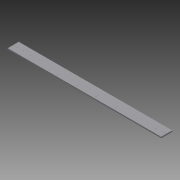
# Autodesk Inventor part: licht_50
Saved by Autodesk Inventor 2015 (Build 190159000, 159)
## iProperties
Created: 2018-01-11
Part Number: licht_50
Material: Generisch
Document SubType Name: Modeling
Designer: schueler
Density: 1 g/cm^3
Appearance: Vorgabe
Author: schueler
Autodesk Inventor part; units mm, degrees
ref_plane "YZ Plane" through (0, 0, 0) normal (1, 0, 0) x (0, 1, 0)
ref_plane "XZ Plane" through (0, 0, 0) normal (0, 1, 0) x (-1, 0, 0)
ref_plane "XY Plane" through (0, 0, 0) normal (0, 0, 1) x (1, 0, 0)
sketch "Skizze1" plane through (0, 0, 0) normal (0, 0, 1) x (1, 0, 0)
  line L0 (0, 0) -> (2000, 0)
  line L1 (2000, 0) -> (2000, 144)
  line L2 (2000, 144) -> (0, 144)
  line L3 (0, 144) -> (0, 0)
  line L4 (0, 25) -> (2000, 25) construction
  line L5 (0, 50) -> (2000, 50) construction
  line L6 (1000, 0) -> (1000, 144) construction
  line L7 (875, 0) -> (875, 144) construction
  line L8 (1125, 144) -> (1125, 0) construction
  line L9 (1375, 144) -> (1375, 0) construction
  line L10 (625, 144) -> (625, 0) construction
  circle A0 centre (625, 50) radius 2.5
  circle A1 centre (875, 50) radius 2.5
  circle A2 centre (1125, 50) radius 2.5
  circle A3 centre (1375, 50) radius 2.5
  circle A4 centre (1375, 25) radius 3.5
  circle A5 centre (1125, 25) radius 3.5
  circle A6 centre (875, 25) radius 3.5
  circle A7 centre (625, 25) radius 3.5
  line L11 (50, 144) -> (50, 0) construction
  circle A8 centre (50, 72) radius 4
  line L12 (1950, 144) -> (1950, 0) construction
  circle A9 centre (1950, 72) radius 4
  line L13 (1992, 144) -> (1992, 0) construction
  line L14 (2000, 112) -> (0, 112) construction
  line L15 (2000, 32) -> (0, 32) construction
  circle A10 centre (1992, 112) radius 1.5
  circle A11 centre (1992, 32) radius 1.5
  line L16 (8, 144) -> (8, 0) construction
  circle A12 centre (8, 112) radius 1.5
  circle A13 centre (8, 72) radius 1.5
  circle A14 centre (8, 32) radius 1.5
  circle A15 centre (1992, 72) radius 1.5
  circle A16 centre (1000, 72) radius 1.5
  circle A17 centre (1000, 112) radius 1.5
  circle A18 centre (1000, 32) radius 1.5
  circle A19 centre (1870, 62) radius 1.5
  circle A20 centre (1970, 72) radius 1.5
  circle A21 centre (1870, 82) radius 1.5
  circle A22 centre (1670, 82) radius 1.5
  circle A23 centre (1670, 62) radius 1.5
  circle A24 centre (1770, 72) radius 1.5
  line L17 (2000, 72) -> (1650, 72) construction
  line L18 (1870, 82) -> (1670, 82) construction
  line L19 (1670, 82) -> (1670, 62) construction
  line L20 (1670, 62) -> (1870, 62) construction
  line L21 (1870, 62) -> (1870, 82) construction
  line L22 (0, 72) -> (350, 72) construction
  circle A25 centre (30, 72) radius 1.5
  circle A26 centre (130, 82) radius 1.5
  circle A27 centre (130, 62) radius 1.5
  circle A28 centre (230, 72) radius 1.5
  circle A29 centre (330, 82) radius 1.5
  circle A30 centre (330, 62) radius 1.5
  line L23 (130, 82) -> (330, 82) construction
  line L24 (330, 82) -> (330, 62) construction
  line L25 (330, 62) -> (130, 62) construction
  line L26 (130, 62) -> (130, 82) construction
  dimension "d0" = 2000
  dimension "d1" = 144
  dimension "d2" = 25
  dimension "d3" = 50
  dimension "d4" = 125
  dimension "d5" = 125
  dimension "d6" = 250
  dimension "d7" = 250
  dimension "d8" = 5
  dimension "d9" = 5
  dimension "d10" = 5
  dimension "d11" = 5
  dimension "d12" = 7
  dimension "d13" = 7
  dimension "d14" = 7
  dimension "d15" = 7
  dimension "d16" = 50
  dimension "d17" = 8
  dimension "d18" = 50
  dimension "d19" = 8
  dimension "d20" = 8
  dimension "d21" = 40
  dimension "d22" = 40
  dimension "d23" = 3
  dimension "d24" = 3
  dimension "d25" = 8
  dimension "d26" = 3
  dimension "d27" = 3
  dimension "d28" = 3
  dimension "d29" = 3
  dimension "d30" = 3
  dimension "d31" = 3
  dimension "d32" = 3
  dimension "d137" = 3
  dimension "d138" = 3
  dimension "d139" = 3
  dimension "d141" = 3
  dimension "d142" = 3
  dimension "d143" = 3
  dimension "d144" = 350
  dimension "d145" = 30
  dimension "d146" = 100
  dimension "d147" = 100
  dimension "d148" = 100
  dimension "d149" = 10
  dimension "d150" = 10
  dimension "d151" = 350
  dimension "d152" = 3
  dimension "d153" = 3
  dimension "d154" = 3
  dimension "d155" = 3
  dimension "d156" = 3
  dimension "d157" = 3
  dimension "d158" = 30
  dimension "d159" = 100
  dimension "d160" = 100
  dimension "d161" = 100
  dimension "d162" = 10
  dimension "d163" = 10
  constraints: 50 end point, 38 point on line, 31 centre point, 9 midpoint, 9 vertical, 6 coincident, 6 parallel, 5 perpendicular, 4 horizontal, 24 other
  measures "d0" distance of L3.start L1.end
  measures "d1" distance of L1.end L1.start
  measures "d2" distance of L1.start L4.end
  measures "d3" distance of L1.start L5.end
  measures "d4" distance of L8.start L6.end
  measures "d5" distance of L7.end L6.end
  measures "d6" distance of L9.start L8.start
  measures "d7" distance of L10.start L7.end
  measures "d8" diameter of A0
  measures "d9" diameter of A1
  measures "d10" diameter of A2
  measures "d11" diameter of A3
  measures "d12" diameter of A4
  measures "d13" diameter of A5
  measures "d14" diameter of A6
  measures "d15" diameter of A7
  measures "d16" distance of L3.start L11.start
  measures "d17" diameter of A8
  measures "d18" distance of L1.end L12.start
  measures "d19" diameter of A9
  measures "d20" distance of L1.end L13.start
  measures "d21" distance of L14.start L17.start
  measures "d22" distance of L15.start L17.start
  measures "d23" diameter of A10
  measures "d24" diameter of A11
  measures "d25" distance of L16.start L3.start
  measures "d26" diameter of A12
  measures "d27" diameter of A13
  measures "d28" diameter of A14
  measures "d29" diameter of A15
  measures "d30" diameter of A16
  measures "d31" diameter of A17
  measures "d32" diameter of A18
  measures "d137" diameter of A19
  measures "d138" diameter of A20
  measures "d139" diameter of A21
  measures "d141" diameter of A22
  measures "d142" diameter of A23
  measures "d143" diameter of A24
  measures "d144" distance of L17.start L17.end
  measures "d145" distance from line of L1 A20.centre
  measures "d146" horizontal distance of L18.start A20.centre
  measures "d147" horizontal distance of A24.centre L18.start
  measures "d148" horizontal distance of A22.centre A24.centre
  measures "d149" distance from line of L17 A22.centre
  measures "d150" distance from line of L17 L19.end
  measures "d151" distance of L22.start L22.end
  measures "d152" diameter of A25
  measures "d153" diameter of A26
  measures "d154" diameter of A27
  measures "d155" diameter of A28
  measures "d156" diameter of A29
  measures "d157" diameter of A30
  measures "d158" distance from line of L3 A25.centre
  measures "d159" distance from line of L26 A25.centre
  measures "d160" distance from line of A28.centre L26
  measures "d161" distance from line of L24 A28.centre
  measures "d162" distance between parallel lines of L22 L23
  measures "d163" distance between parallel lines of L25 L22
extrude "Extrusion1" add sketch "Skizze1" along normal blind 16
hole "Bohrung1" at (1375, 25, 0) at (1125, 25, 0) at (875, 25, 0) at (625, 25, 0) direction (0, 0, 1) diameter 10 depth 12 tip angle 118
hole "Bohrung4" at (1125, 50, 0) at (875, 50, 0) at (625, 50, 0) at (1375, 50, 0) direction (0, 0, 1) diameter 7 depth 12 tip angle 118
sketch "Skizze4" plane through (0, 0, 16) normal (0, 0, 1) x (1, 0, 0)
  circle A0 centre (8, 112) radius 1.5 projected
  circle A1 centre (8, 72) radius 1.5 projected
  circle A2 centre (8, 32) radius 1.5 projected
  circle A3 centre (30, 72) radius 1.5 projected
  circle A4 centre (1950, 72) radius 4 projected
  circle A5 centre (50, 72) radius 4 projected
  circle A6 centre (625, 25) radius 3.5 projected
  circle A7 centre (875, 25) radius 3.5 projected
  circle A8 centre (1125, 25) radius 3.5 projected
  circle A9 centre (1375, 25) radius 3.5 projected
  circle A10 centre (1375, 50) radius 2.5 projected
  circle A11 centre (1125, 50) radius 2.5 projected
  circle A12 centre (875, 50) radius 2.5 projected
  circle A13 centre (625, 50) radius 2.5 projected
  circle A14 centre (330, 62) radius 1.5 projected
  circle A15 centre (330, 82) radius 1.5 projected
  circle A16 centre (230, 72) radius 1.5 projected
  circle A17 centre (130, 62) radius 1.5 projected
  circle A18 centre (130, 82) radius 1.5 projected
  circle A19 centre (30, 72) radius 1.5 projected
  circle A20 centre (1770, 72) radius 1.5 projected
  circle A21 centre (1670, 62) radius 1.5 projected
  circle A22 centre (1670, 82) radius 1.5 projected
  circle A23 centre (1870, 82) radius 1.5 projected
  circle A24 centre (1970, 72) radius 1.5 projected
  circle A25 centre (1870, 62) radius 1.5 projected
  circle A26 centre (1000, 32) radius 1.5 projected
  circle A27 centre (1000, 112) radius 1.5 projected
  circle A28 centre (1000, 72) radius 1.5 projected
  circle A29 centre (1992, 72) radius 1.5 projected
  circle A30 centre (8, 32) radius 1.5 projected
  circle A31 centre (8, 72) radius 1.5 projected
  circle A32 centre (8, 112) radius 1.5 projected
  circle A33 centre (1992, 32) radius 1.5 projected
  circle A34 centre (1992, 112) radius 1.5 projected
  line L0 (0, 0) -> (2000, 0) projected
  line L1 (2000, 0) -> (2000, 144) projected
  line L2 (2000, 144) -> (0, 144) projected
  line L3 (0, 144) -> (0, 0) projected
hole "Bohrung15" at (1970, 72, 16) at (1992, 32, 16) at (1992, 72, 16) at (1992, 112, 16) at (1870, 82, 16) at (1870, 62, 16) at (1670, 62, 16) at (1670, 82, 16) at (1770, 72, 16) at (1000, 112, 16) at (1000, 72, 16) at (1000, 32, 16) at (330, 62, 16) at (330, 82, 16) at (230, 72, 16) at (130, 62, 16) at (130, 82, 16) at (8, 72, 16) at (8, 72, 16) at (30, 72, 16) at (30, 72, 16) at (8, 112, 16) at (8, 112, 16) at (8, 32, 16) at (8, 32, 16) direction (0, 0, -1) diameter 3 depth 8 tip angle 118 countersink diameter 8 countersink angle 90
sketch "Skizze5" plane through (0, 144, 0) normal (0, 1, 0) x (1, 0, 0)
  line L0 (2000, -16) -> (0, -16) construction
  line L1 (0, -16) -> (0, 0) construction
  line L2 (0, 0) -> (2000, 0) construction
  line L3 (2000, 0) -> (2000, -16) construction
  line L4 (0, 0) -> (0, -16) construction
  line L5 (0, -8) -> (2000, -8) construction
  line L6 (2000, 0) -> (2000, -16) construction
  line L7 (0, -16) -> (2000, -16) construction
  line L8 (1000, -16) -> (1000, 0) construction
  line L9 (0, 0) -> (2000, 0) construction
  point P0 (1100, -8)
  point P1 (1300, -8)
  point P2 (1500, -8)
  point P3 (1700, -8)
  point P4 (1900, -8)
  point P5 (900, -8)
  point P6 (700, -8)
  point P7 (500, -8)
  point P8 (300, -8)
  point P9 (100, -8)
  dimension "d189" = 100
  dimension "d190" = 200
  dimension "d191" = 200
  dimension "d192" = 200
  dimension "d193" = 200
  dimension "d194" = 100
  dimension "d195" = 200
  dimension "d196" = 200
  dimension "d197" = 200
  dimension "d198" = 200
  constraints: 10 end point, 4 midpoint, 2 parallel, 1 horizontal, 1 perpendicular, 13 other
  measures "d189" horizontal distance of point (900, -8) L8.start
  measures "d190" distance of point (700, -8) point (900, -8)
  measures "d191" distance of point (500, -8) point (700, -8)
  measures "d192" distance of point (300, -8) point (500, -8)
  measures "d193" distance of point (300, -8) point (100, -8)
  measures "d194" distance from line of L8 point (1100, -8)
  measures "d195" distance of point (1100, -8) point (1300, -8)
  measures "d196" distance of point (1300, -8) point (1500, -8)
  measures "d197" distance of point (1500, -8) point (1700, -8)
  measures "d198" distance of point (1700, -8) point (1900, -8)
hole "Bohrung16" at (1900, 144, 8) at (1700, 144, 8) at (1500, 144, 8) at (1300, 144, 8) at (900, 144, 8) at (700, 144, 8) at (500, 144, 8) at (1100, 144, 8) at (300, 144, 8) at (100, 144, 8) direction (0, -1, 0) diameter 3 depth 30 tip angle 118
